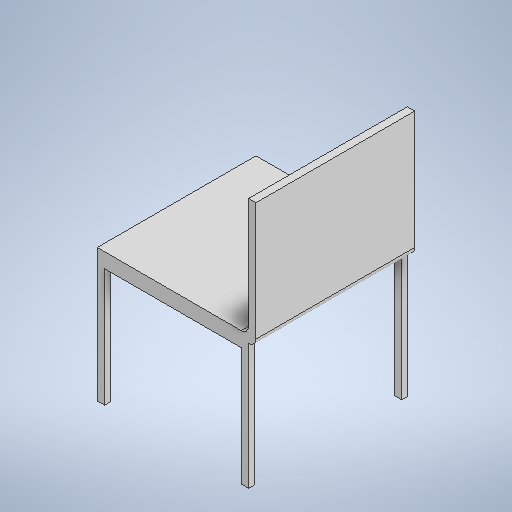
# Autodesk Inventor part: chair
Saved by Autodesk Inventor 2027 (Build 310192000, 192)
## iProperties
Created: 2026-05-26
Part Number: chair
Material: Generic
Document SubType Name: Modeling
Designer: cheap
Density: 1 g/cm^3
Appearance: Default
Author: cheap
Autodesk Inventor part; units mm, degrees
ref_plane "YZ Plane" through (0, 0, 0) normal (1, 0, 0) x (0, 1, 0)
ref_plane "XZ Plane" through (0, 0, 0) normal (0, 1, 0) x (-1, 0, 0)
ref_plane "XY Plane" through (0, 0, 0) normal (0, 0, 1) x (1, 0, 0)
sketch "Sketch1" plane through (0, 0, 0) normal (0, 0, 1) x (1, 0, 0)
  line L0 (-25.4, 0) -> (-520.7, 0)
  line L1 (0, 25.4) -> (0, 406.4)
  line L2 (25.4, 406.4) -> (25.4, 0)
  line L3 (0, -25.4) -> (-520.7, -25.4)
  line L4 (-520.7, 0) -> (-520.7, -25.4)
  line L5 (25.4, 406.4) -> (0, 406.4)
  arc A0 (22.225, -25.4) -> (25.4, -22.225) centre (22.225, -22.225) ccw
  arc A1 (-25.4, 0) -> (0, 25.4) centre (-25.4, 25.4) ccw
  arc A2 (0, -25.4) -> (25.4, 0) centre (0, 0) ccw
  point P0 (0, 0)
  dimension "d0" = 520.7
  dimension "d1" = 406.4
  dimension "d2" = 25.4
  dimension "d3" = 3.175
  dimension "d6" = 25.4
  constraints: 12 end point, 6 point on circle, 6 tangent, 4 point on line, 3 centre point, 2 vertical, 1 equal radius, 1 horizontal, 1 perpendicular, 1 other
  measures "d0" distance of point (0, 0) L0.end
  measures "d1" distance of point (0, 0) L1.end
  measures "d2" distance between parallel lines of L1 L2
  measures "d3" radius of A0
  measures "d6" radius of A1
extrude "Extrusion1" add sketch "Sketch1" along normal blind 546.1
sketch "Sketch2" plane through (-520.7, -25.4, 0) normal (0, -1, 0) x (1, 0, 0)
  line L0 (520.7, 0) -> (520.7, 546.1) construction
  line L1 (520.7, 273.05) -> (0, 273.05) construction
  line L2 (0, 0) -> (0, 546.1) construction
  line L3 (495.3, 546.1) -> (0, 546.1) construction
  line L4 (260.35, 546.1) -> (260.35, 0) construction
  line L5 (0, 0) -> (520.7, 0) construction
  line L6 (495.3, 546.1) -> (495.3, 527.05)
  line L7 (495.3, 0) -> (495.3, 546.1) projected
  line L8 (495.3, 527.05) -> (25.4, 527.05)
  line L9 (25.4, 527.05) -> (25.4, 546.1)
  line L10 (495.3, 546.1) -> (25.4, 546.1)
  line L11 (495.3, 0) -> (0, 0) construction
  line L12 (495.3, 0) -> (495.3, 19.05)
  line L13 (495.3, 19.05) -> (25.4, 19.05)
  line L14 (25.4, 19.05) -> (25.4, 0)
  line L15 (495.3, 0) -> (25.4, 0)
  point P0 (25.4, 536.575)
  point P1 (25.4, 9.525)
  dimension "d7" = 19.05
  dimension "d8" = 25.4
  constraints: 22 end point, 5 point on line, 4 midpoint, 4 symmetric about line, 2 horizontal, 1 perpendicular
  measures "d7" distance of L3.start L6.end
  measures "d8" distance from line of L2 point (25.4, 536.575)
extrude "Extrusion2" add sketch "Sketch2" along normal blind 25.4
sketch "Sketch4" plane through (0, -25.4, 0) normal (0, -1, 0) x (1, 0, 0)
  line L0 (-25.4, 527.05) -> (-25.4, 546.1) projected
  line L1 (-25.4, 527.05) -> (0, 527.05)
  line L2 (0, 0) -> (0, 546.1) projected
  line L3 (-25.4, 546.1) -> (-495.3, 546.1) projected
  line L4 (0, 546.1) -> (-25.4, 546.1)
  line L5 (-25.4, 546.1) -> (-25.4, 527.05)
  line L6 (25.4, 0) -> (25.4, 546.1) construction
  line L7 (25.4, 273.05) -> (-520.7, 273.05) construction
  line L8 (-520.7, 0) -> (-520.7, 546.1) construction
  line L9 (-495.3, 0) -> (-25.4, 0) construction
  line L10 (-247.65, 0) -> (-247.65, 546.1) construction
  line L11 (-25.4, 19.05) -> (-25.4, 0)
  line L12 (-25.4, 19.05) -> (0, 19.05)
  line L13 (0, 0) -> (-25.4, 0)
  line L14 (-25.4, 0) -> (-25.4, 19.05)
  line L15 (-495.3, 546.1) -> (-520.7, 546.1)
  line L16 (-520.7, 527.05) -> (-495.3, 527.05)
  line L17 (-495.3, 527.05) -> (-495.3, 546.1)
  line L18 (-495.3, 0) -> (-495.3, 19.05) projected
  line L19 (-495.3, 19.05) -> (-520.7, 19.05)
  line L20 (-520.7, 0) -> (-495.3, 0) projected
  line L21 (-520.7, 0) -> (-495.3, 0)
  line L22 (-495.3, 0) -> (-495.3, 19.05)
  line L23 (-25.4, 546.1) -> (-25.4, 527.05)
  line L24 (0, 546.1) -> (0, 527.05)
  line L25 (-495.3, 546.1) -> (-495.3, 527.05)
  line L26 (-520.7, 527.05) -> (-520.7, 546.1)
  line L27 (-495.3, 19.05) -> (-495.3, 0)
  line L28 (-520.7, 0) -> (-520.7, 19.05)
  constraints: 42 end point, 7 perpendicular, 5 point on line, 3 collinear, 3 horizontal, 2 midpoint, 2 parallel, 2 symmetric about line, 1 vertical
extrude "Extrusion3" add sketch "Sketch4" along normal blind 431.8
body "Solid1"
